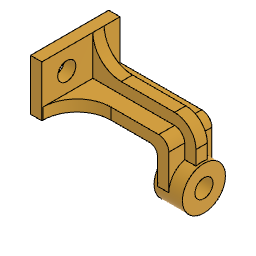
Figure-8 (Autodesk Fusion 360 design; units mm, degrees)
Autodesk Fusion 360 part; units mm, degrees
sketch "Sketch1" plane through (0, 0, 0) normal (1, 0, 0) x (0, 1, 0)
  circle A0 centre (0, 0) radius 19
  dimension "d1" = 38
  constraint coincident A0.centre origin
  measures "d1" diameter of A0
extrude "Extrude1" add sketch "Sketch1" along normal blind 25
sketch "Sketch2" plane through (0, 0, 0) normal (0, 1, 0) x (1, 0, 0)
  line L0 (23, 0) -> (23, -31.0562)
  arc A0 (4.0562, -50) -> (23, -31.0562) centre (4.0562, -31.0562) ccw
  line L1 (4.0562, -50) -> (-68, -50)
  line L2 (-68, -50) -> (-68, -40)
  line L3 (-68, -40) -> (4.0562, -40)
  arc A1 (4.0562, -40) -> (13, -31.0562) centre (4.0562, -31.0562) ccw
  line L4 (13, -31.0562) -> (13, 0)
  line L5 (13, 0) -> (23, 0)
  line L6 (25, -19) -> (25, 19)
  dimension "d4" = 2
  dimension "d5" = 91
  dimension "d6" = 50
  dimension "d7" = 10
  constraint vertical L0
  constraint tangent L0 A0
  constraint tangent A0 L1
  constraint perpendicular L0 L1
  constraint perpendicular L1 L2
  constraint perpendicular L2 L3
  constraint tangent L3 A1
  constraint perpendicular L3 L4
  constraint perpendicular L0 L5
  constraint tangent A1 L4
  constraint concentric A0 A1
  measures "d4" distance of L0 L6
  measures "d5" horizontal distance of L0.start L2.end
  measures "d6" vertical distance of L0.start A0.start
  measures "d7" distance of L1.end L2.end
extrude "Extrude2" add sketch "Sketch2" along normal mid plane 10
sketch "Sketch4" plane through (0, 0, 0) normal (0, 1, 0) x (1, 0, 0)
  line L0 (13, 0) -> (13, -31.0562)
  arc A0 (4.0562, -40) -> (13, -31.0562) centre (4.0562, -31.0562) ccw
  line L1 (4.0562, -40) -> (-68, -40)
  line L2 (-68, -40) -> (-68, -30)
  line L3 (-68, -30) -> (-3.8, -30)
  arc A1 (-3.8, -30) -> (3, -23.2) centre (-3.8, -23.2) ccw
  line L4 (3, -23.2) -> (3, 0)
  line L5 (3, 0) -> (13, 0)
  line L6 (-68, -40) -> (4.0562, -40)
  line L7 (13, -31.0562) -> (13, -18.3303)
  arc A2 (4.0562, -40) -> (13, -31.0562) centre (4.0562, -31.0562) ccw
  constraint vertical L0
  constraint tangent L0 A0
  constraint perpendicular L0 L1
  constraint perpendicular L1 L2
  constraint perpendicular L2 L3
  constraint tangent L3 A1
  constraint perpendicular L1 L4
  constraint perpendicular L0 L5
  constraint collinear L1 L6
  constraint collinear L0 L7
  constraint coincident L2 L1.end
  constraint coincident origin L5
  constraint tangent A0 L1
  constraint tangent A1 L4
  constraint concentric A0 A2
extrude "Extrude3" add sketch "Sketch4" along normal mid plane 38
sketch "Sketch5" plane through (0, 0, 0) normal (1, 0, 0) x (0, 1, 0)
  line L0 (19, 30, -68) -> (-50, 30, -68)
  line L1 (-50, 30, -68) -> (-50, 75, -68)
  line L2 (-50, 75, -68) -> (19, 75, -68)
  line L3 (19, 75, -68) -> (19, 30, -68)
  point P0 (19, 30)
  dimension "d20" = 69
  dimension "d21" = 45
extrude "Extrude4" add sketch "Sketch5" against normal blind 10 contours L0 L1 L2 L3 in plane through (-68, 0, 0) normal (1, 0, 0)
fillet "Fillet1" radius 25 1 edges at (-68, 0, 50)
fillet "Fillet2" radius 30 1 edges at (-68, -19, 35)
sketch "Sketch7" plane through (0, 0, 0) normal (1, 0, 0) x (0, 1, 0)
  circle A0 through (8, 0, 25) (-4, 6.9282, 25) (-4, -6.9282, 25)
  dimension "d29" = 16
extrude "Extrude5" cut sketch "Sketch7" against normal blind 175 contours A0 in plane through (25, 0, 0) normal (1, 0, 0)
sketch "Sketch9" plane through (-68, 0, 0) normal (1, 0, 0) x (0, 1, 0)
  line L0 (-49, 30) -> (-49, 40)
  line L1 (-49, 40) -> (-5, 40)
  line L2 (-5, 40) -> (-5, 75)
  line L3 (-5, 75) -> (-50, 75)
  line L4 (-50, 75) -> (-50, 30)
  line L5 (-50, 30) -> (-49, 30)
  circle A0 centre (-28, 57) radius 8
  dimension "d32" = 16
  dimension "d33" = 22
  dimension "d34" = 18
  measures "d32" diameter of A0
  measures "d33" distance of L4 A0.centre
  measures "d34" distance of L3 A0.centre
extrude "Extrude6" cut sketch "Sketch9" against normal blind 80 contours A0
